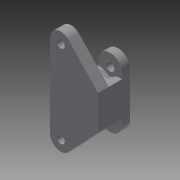
# Autodesk Inventor part: TestMount
Saved by Autodesk Inventor 2015 (Build 190159000, 159)
## iProperties
Created: 2017-03-05
Part Number: TestMount
Material: Generic
Document SubType Name: Modeling
Designer: 1esh9
Density: 1 g/cm^3
Appearance: Default
Author: 1esh9
Autodesk Inventor part; units mm, degrees
ref_plane "YZ Plane" through (0, 0, 0) normal (1, 0, 0) x (0, 1, 0)
ref_plane "XZ Plane" through (0, 0, 0) normal (0, 1, 0) x (-1, 0, 0)
ref_plane "XY Plane" through (0, 0, 0) normal (0, 0, 1) x (1, 0, 0)
sketch "Sketch1" plane through (0, 0, 0) normal (0, 1, 0) x (-1, 0, 0)
  circle A0 centre (5.65, 15.5) radius 1.5
  circle A1 centre (5.65, -15.5) radius 1.5
  circle A2 centre (5.65, 15.5) radius 4
  circle A3 centre (5.65, -15.5) radius 4
  line L0 (-8.345, 6.5) -> (-8.345, -6.5)
  line L1 (5.65, 15.5) -> (5.65, -15.5) construction
  line L2 (9.65, 15.5) -> (9.65, -15.5)
  line L3 (-8.345, 6.5) -> (2.7411, 18.2456)
  line L4 (-8.345, -6.5) -> (2.7411, -18.2456)
  line L5 (-8.345, 6.5) -> (0.605, 6.5)
  line L6 (0.605, 6.5) -> (0.605, -6.5)
  line L7 (0.605, -6.5) -> (-8.345, -6.5)
  line L8 (-8.345, -6.5) -> (-8.345, 6.5)
  point P0 (0, 0)
  dimension "d0" = 31
  dimension "d1" = 15.5
  dimension "d2" = 3
  dimension "d3" = 3
  dimension "d4" = 5.65
  dimension "d5" = 5.65
  dimension "d6" = 8
  dimension "d7" = 8
  dimension "d8" = 8.345
  dimension "d11" = 13
  dimension "d12" = 6.5
  dimension "d13" = 0.605
  constraints: 18 end point, 4 centre point, 4 point on circle, 3 tangent, 2 coincident, 2 parallel, 1 horizontal, 1 perpendicular, 1 vertical
  measures "d0" distance of A1.centre A0.centre
  measures "d1" vertical distance of point (0, 0) A0.centre
  measures "d2" diameter of A0
  measures "d3" diameter of A1
  measures "d4" horizontal distance of point (0, 0) A0.centre
  measures "d5" horizontal distance of point (0, 0) A1.centre
  measures "d6" diameter of A2
  measures "d7" diameter of A3
  measures "d8" distance from line of point (0, 0) L0
  measures "d11" distance of L0.start L0.end
  measures "d12" vertical distance of point (0, 0) L0.start
  measures "d13" distance from line of point (0, 0) L6
extrude "Extrusion1" add sketch "Sketch1" along normal blind 4 contours A2 | L2 A3 L4 L7 L6 L5 L3 A2 | A3
extrude "Extrusion2" add sketch "Sketch1" along normal blind 8.96 contours L5 L6 L7 L0
sketch "Sketch2" plane through (0, 8.96, 0) normal (0, 1, 0) x (1, 0, 0)
  line L0 (8.345, -6.5) -> (8.345, 6.5) projected
  line L1 (8.345, 6.5) -> (-0.605, 6.5) projected
  line L2 (-0.605, 6.5) -> (-0.605, -6.5) projected
  line L3 (-0.605, -6.5) -> (8.345, -6.5) projected
  circle A0 centre (3.87, -8.4) radius 1.6
  circle A1 centre (3.87, 8.4) radius 1.6
  arc A2 (-0.605, -8.4) -> (8.345, -8.4) centre (3.87, -8.4) ccw
  arc A3 (8.345, 8.4) -> (-0.605, 8.4) centre (3.87, 8.4) ccw
  line L4 (-0.605, -8.4) -> (-0.605, 8.4)
  line L5 (8.345, 8.4) -> (8.345, -8.4)
  point P0 (0, 0)
  dimension "d18" = 8.95
  dimension "d19" = 4.475
  dimension "d20" = 4.475
  dimension "d21" = 16.8
  dimension "d22" = 8.4
  dimension "d23" = 8.95
  dimension "d24" = 3.2
  dimension "d25" = 3.2
  constraints: 4 centre point, 4 end point, 4 point on circle, 3 tangent, 2 coincident
  measures "d18" distance of L2.end L0.start
  measures "d19" distance from line of L0 A0.centre
  measures "d20" distance from line of L0 A1.centre
  measures "d21" distance of A1.centre A0.centre
  measures "d22" vertical distance of point (0, 0) A0.centre
  measures "d23" diameter of A2
  measures "d24" diameter of A0
  measures "d25" diameter of A1
extrude "Extrusion3" add sketch "Sketch2" along normal blind 3
sketch "Sketch3" plane through (0, 8.96, 0) normal (0, -1, 0) x (1, 0, 0)
  circle A0 centre (3.87, 8.4) radius 1.6 projected
  circle A1 centre (3.87, 8.4) radius 1.6 projected
  circle A2 centre (3.87, -8.4) radius 1.6 projected
  circle A3 centre (3.87, -8.4) radius 1.6 projected
  line L0 (3.87, 4.9359) -> (0.87, 6.6679)
  line L1 (0.87, 6.6679) -> (0.87, 10.1321)
  line L2 (0.87, 10.1321) -> (3.87, 11.8641)
  line L3 (3.87, 11.8641) -> (6.87, 10.1321)
  line L4 (6.87, 10.1321) -> (6.87, 6.6679)
  line L5 (6.87, 6.6679) -> (3.87, 4.9359)
  line L6 (3.87, -4.9359) -> (6.87, -6.6679)
  line L7 (6.87, -6.6679) -> (6.87, -10.1321)
  line L8 (6.87, -10.1321) -> (3.87, -11.8641)
  line L9 (3.87, -11.8641) -> (0.87, -10.1321)
  line L10 (0.87, -10.1321) -> (0.87, -6.6679)
  line L11 (0.87, -6.6679) -> (3.87, -4.9359)
  point P0 (0, 0)
  dimension "d28" = 6
  dimension "d29" = 6
  constraints: 24 end point, 2 coincident, 26 other
  measures "d28" distance between parallel lines of L4 L1
  measures "d29" distance between parallel lines of L10 L7
extrude "Extrusion4" cut sketch "Sketch3" along normal blind 2.5
equation "\"d1\" = 0.5 * d0"
equation "\"d12\" = 0.5 * d11"
equation "\"d19\" = 0.5 * d18"
equation "\"d20\" = 0.5 * d18"
equation "\"d22\" = 0.5 * d21"
body "Solid1"
